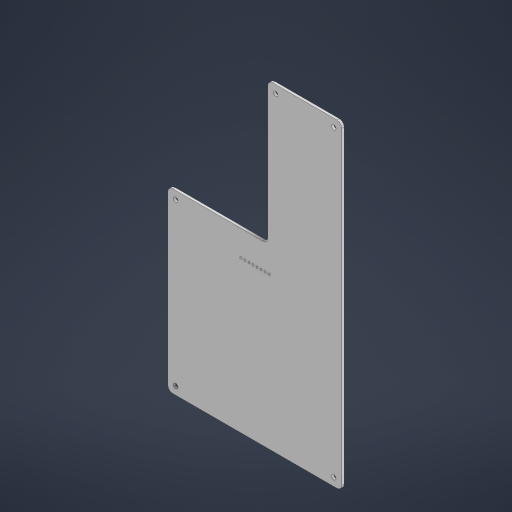
# Autodesk Inventor part: Motherboard
Saved by Autodesk Inventor 2023 (Build 270158000, 158)
## iProperties
Created: 2023-07-12
Part Number: Motherboard
Material: Типовые
Document SubType Name: Modeling
Designer: khrip
Density: 1 g/cm^3
Appearance: По умолчанию
Author: khrip
Autodesk Inventor part; units mm, degrees
ref_plane "YZ Plane" through (0, 0, 0) normal (1, 0, 0) x (0, 1, 0)
ref_plane "XZ Plane" through (0, 0, 0) normal (0, 1, 0) x (-1, 0, 0)
ref_plane "XY Plane" through (0, 0, 0) normal (0, 0, 1) x (1, 0, 0)
ref_plane "РабПлоскость1" through (0, 0, 0) normal (0, 0, 1) x (1, 0, 0)
ref_plane "РабПлоскость2" through (0, 0, 0) normal (0, 0, 1) x (1, 0, 0)
sketch "Эскиз2" plane through (0, 0, 0) normal (0, 0, 1) x (1, 0, 0)
  line L0 (164.5082, 55.3787) -> (164.5082, 22.6213)
  line L1 (152.0082, 55.3787) -> (164.5082, 55.3787)
  spline S0 degree 4 poles (142.0082, 66.7804) (141.9936, 65.5806) (142.2897, 63.8407) (143.0904, 61.8123) (144.7867, 59.6039) (146.7684, 57.7973) (148.9036, 56.5519) (150.6395, 55.9298) (152.0082, 55.3787) knots 0 0 0 0 0 0.305903 0.428365 0.551581 0.676311 1 1 1 1 1
  line L2 (142.0082, 89.6988) -> (142.0082, 66.7804)
  spline S1 degree 4 poles (142.0976, 90.5077) (142.1863, 90.3272) (142.1406, 90.1079) (142.065, 89.9075) (142.0082, 89.6988) knots 0 0 0 0 0 1 1 1 1 1
  ellipse E0 centre (144.0082, 89.6716) end of major axis (144.0082, 92.5) minor radius 2 (144.0082, 92.5) -> (142.0976, 90.5077) ccw
  line L3 (144.0082, 92.5) -> (149.4338, 92.5)
  line L4 (149.4338, 92.5) -> (149.4338, 92.525)
  line L5 (149.4338, 92.525) -> (142.946, 92.525)
  ellipse E1 centre (142.946, 98.525) end of major axis (136.7344, 98.525) minor radius 6 (136.7344, 98.525) -> (142.946, 92.525) ccw
  line L6 (136.7344, 98.525) -> (136.7344, 100.025)
  ellipse E2 centre (142.946, 100.025) end of major axis (136.7344, 100.025) minor radius 6 (142.946, 106.025) -> (136.7344, 100.025) ccw
  line L7 (142.946, 106.025) -> (149.4338, 106.025)
  line L8 (149.4338, 106.025) -> (149.4338, 106.05)
  line L9 (149.4338, 106.05) -> (144.0082, 106.05)
  ellipse E3 centre (144.0082, 108.8784) end of major axis (144.0082, 106.05) minor radius 2 (142.0976, 108.0423) -> (144.0082, 106.05) ccw
  spline S2 degree 4 poles (142.0082, 108.8512) (142.0222, 108.6489) (142.0418, 108.4466) (142.067, 108.2444) (142.0976, 108.0423) knots 0 0 0 0 0 1 1 1 1 1
  line L10 (142.0082, 108.8512) -> (142.0082, 139)
  arc A0 (142.0082, 139) -> (137.0082, 144) centre (137.0082, 139) ccw
  line L11 (137.0082, 144) -> (27.0082, 144)
  arc A1 (27.0082, 144) -> (22.0082, 139) centre (27.0082, 139) ccw
  line L12 (22.0082, 139) -> (22.0082, 108.8512)
  spline S3 degree 4 poles (21.9188, 108.0423) (21.9596, 108.2417) (21.9876, 108.4433) (22.0035, 108.6467) (22.0082, 108.8512) knots 0 0 0 0 0 1 1 1 1 1
  ellipse E4 centre (20.0082, 108.8784) end of major axis (20.0082, 106.05) minor radius 2 (20.0082, 106.05) -> (21.9188, 108.0423) ccw
  line L13 (14.5826, 106.05) -> (20.0082, 106.05)
  line L14 (14.5826, 106.025) -> (14.5826, 106.05)
  line L15 (21.0704, 106.025) -> (14.5826, 106.025)
  ellipse E5 centre (21.0704, 100.025) end of major axis (27.282, 100.025) minor radius 6 (27.282, 100.025) -> (21.0704, 106.025) ccw
  ellipse E6 centre (21.0704, 98.525) end of major axis (27.282, 98.525) minor radius 6 (21.0704, 92.525) -> (27.282, 98.525) ccw
  line L16 (14.5826, 92.525) -> (21.0704, 92.525)
  line L17 (14.5826, 92.5) -> (14.5826, 92.525)
  line L18 (20.0082, 92.5) -> (14.5826, 92.5)
  ellipse E7 centre (20.0082, 89.6716) end of major axis (20.0082, 92.5) minor radius 2 (21.9188, 90.5077) -> (20.0082, 92.5) ccw
  spline S4 degree 4 poles (22.0082, 89.6988) (22.0001, 89.9001) (21.9823, 90.1037) (21.9553, 90.3071) (21.9188, 90.5077) knots 0 0 0 0 0 1 1 1 1 1
  line L19 (22.0082, 89.6988) -> (22.0082, 66.7804)
  spline S5 degree 4 poles (12.0082, 55.3787) (13.3543, 55.9133) (15.0972, 56.5843) (17.1914, 57.7632) (19.2093, 59.6353) (20.8508, 61.7502) (21.742, 63.9004) (21.9889, 65.5297) (22.0082, 66.7804) knots 0 0 0 0 0 0.323057 0.447569 0.570948 0.693515 1 1 1 1 1
  line L20 (-0.4918, 55.3787) -> (12.0082, 55.3787)
  line L21 (-0.4918, 22.6213) -> (-0.4918, 55.3787)
  line L22 (12.0082, 22.6213) -> (-0.4918, 22.6213)
  spline S6 degree 4 poles (22.0082, 11.2196) (21.9907, 12.4712) (21.7455, 14.1022) (20.8556, 16.2534) (19.2129, 18.3699) (17.1941, 20.2411) (15.0987, 21.4185) (13.3552, 22.0877) (12.0082, 22.6213) knots 0 0 0 0 0 0.306528 0.4291 0.552475 0.676977 1 1 1 1 1
  line L23 (22.0082, -11.6988) -> (22.0082, 11.2196)
  spline S7 degree 4 poles (22.2969, -12.5077) (22.2375, -12.3039) (22.1691, -12.101) (22.0924, -11.8993) (22.0082, -11.6988) knots 0 0 0 0 0 1 1 1 1 1
  ellipse E8 centre (20.3863, -11.6716) end of major axis (20.3863, -14.5) minor radius 2 (20.3863, -14.5) -> (22.2969, -12.5077) ccw
  line L24 (20.3863, -14.5) -> (14.9607, -14.5)
  line L25 (14.9607, -14.5) -> (14.9607, -14.525)
  line L26 (14.9607, -14.525) -> (21.4484, -14.525)
  ellipse E9 centre (21.4484, -20.525) end of major axis (27.6601, -20.525) minor radius 6 (27.6601, -20.525) -> (21.4484, -14.525) ccw
  line L27 (27.6601, -20.525) -> (27.6601, -22.025)
  ellipse E10 centre (21.4484, -22.025) end of major axis (27.6601, -22.025) minor radius 6 (21.4484, -28.025) -> (27.6601, -22.025) ccw
  line L28 (21.4484, -28.025) -> (14.9607, -28.025)
  line L29 (14.9607, -28.025) -> (14.9607, -28.05)
  line L30 (14.9607, -28.05) -> (20.3863, -28.05)
  ellipse E11 centre (20.3863, -30.8784) end of major axis (20.3863, -28.05) minor radius 2 (22.2969, -30.0423) -> (20.3863, -28.05) ccw
  spline S8 degree 4 poles (22.0082, -30.8512) (22.0994, -30.6437) (22.1874, -30.4372) (22.2667, -30.2332) (22.2969, -30.0423) knots 0 0 0 0 0 1 1 1 1 1
  line L31 (22.0082, -30.8512) -> (22.0082, -61)
  arc A2 (22.0082, -61) -> (27.0082, -66) centre (27.0082, -61) ccw
  line L32 (27.0082, -66) -> (137.0082, -66)
  arc A3 (137.0082, -66) -> (142.0082, -61) centre (137.0082, -61) ccw
  line L33 (142.0082, -61) -> (142.0082, -30.8512)
  spline S9 degree 4 poles (142.0976, -30.0423) (142.0618, -30.2424) (142.0345, -30.444) (142.0164, -30.6471) (142.0082, -30.8512) knots 0 0 0 0 0 1 1 1 1 1
  ellipse E12 centre (144.0082, -30.8784) end of major axis (144.0082, -28.05) minor radius 2 (144.0082, -28.05) -> (142.0976, -30.0423) ccw
  line L34 (149.4338, -28.05) -> (144.0082, -28.05)
  line L35 (149.4338, -28.025) -> (149.4338, -28.05)
  line L36 (142.946, -28.025) -> (149.4338, -28.025)
  ellipse E13 centre (142.946, -22.025) end of major axis (136.7344, -22.025) minor radius 6 (136.7344, -22.025) -> (142.946, -28.025) ccw
  line L37 (136.7344, -20.525) -> (136.7344, -22.025)
  ellipse E14 centre (142.946, -20.525) end of major axis (136.7344, -20.525) minor radius 6 (142.0082, -14.5938) -> (136.7344, -20.525) ccw
  spline S10 degree 4 poles (143.3575, -14.5382) (143.017, -14.5392) (142.6788, -14.5494) (142.3414, -14.5663) (142.0082, -14.5938) knots 0 0 0 0 0 1 1 1 1 1
  spline S11 degree 4 poles (143.3575, -14.5382) (143.1143, -14.3292) (142.8382, -14.0321) (142.6629, -13.7922) (142.4735, -13.4852) knots 0 0 0 0 0 1 1 1 1 1
  ellipse E15 centre (144.0082, -11.6716) end of major axis (144.0082, -8.8431) minor radius 2 (142.0976, -12.5077) -> (142.4735, -13.4852) ccw
  spline S12 degree 4 poles (142.0976, -12.5077) (142.0566, -12.3073) (142.0277, -12.1043) (142.0113, -11.9008) (142.0082, -11.6988) knots 0 0 0 0 0 1 1 1 1 1
  line L38 (142.0082, 11.2196) -> (142.0082, -11.6988)
  spline S13 degree 4 poles (152.0082, 22.6213) (150.6678, 22.0949) (148.9359, 21.4381) (146.8415, 20.2599) (144.8098, 18.3825) (143.1469, 16.2574) (142.2323, 14.098) (142.0013, 12.4654) (142.0082, 11.2196) knots 0 0 0 0 0 0.322163 0.446837 0.570623 0.693583 1 1 1 1 1
  line L39 (164.5082, 22.6213) -> (152.0082, 22.6213)
  line L40 (27.282, 98.525) -> (27.282, 100.025)
  line L41 (27.6601, -66) -> (136.7344, -66)
  line L42 (136.7344, -66) -> (136.7344, 55.12)
  line L43 (85.3082, 55.12) -> (27.6601, 55.12)
  line L44 (27.6601, 55.12) -> (27.6601, -66)
  line L45 (49.6082, 55.12) -> (60.6082, 55.12) projected
  line L46 (85.3082, 55.12) -> (85.3082, 144)
  line L47 (85.3082, 144) -> (136.7344, 144)
  line L48 (136.7344, 144) -> (136.7344, 55.12)
  line L49 (85.3082, 113.52) -> (85.3082, 107.52) projected
  line L50 (84.3244, 70.87) -> (84.3244, 64.87) projected
  line L51 (27.6601, 50.12) -> (90.3082, 50.12)
  line L52 (136.7344, 57.0858) -> (136.7344, -61)
  line L53 (136.7344, -61) -> (27.6601, -61)
  line L54 (27.6601, -61) -> (27.6601, 50.12)
  line L55 (90.3082, 50.12) -> (90.3082, 139)
  line L56 (90.3082, 139) -> (136.7344, 139)
  line L57 (136.7344, 139) -> (136.7344, 57.0858)
  point P0 (0, 0)
  point P1 (142.0243, 108.6495)
  point P2 (142.0445, 108.4475)
  point P3 (142.069, 108.2451)
  point P4 (21.9548, 108.2422)
  point P5 (21.9815, 108.4436)
  point P6 (21.9992, 108.6466)
  point P7 (21.9966, 89.8995)
  point P8 (21.9778, 90.1023)
  point P9 (21.9518, 90.3056)
  point P10 (14.1516, 56.2573)
  point P11 (16.0588, 57.2184)
  point P12 (17.7454, 58.3637)
  point P13 (19.1678, 59.6884)
  point P14 (20.3459, 61.2222)
  point P15 (21.2579, 62.9881)
  point P16 (21.8122, 64.8416)
  point P17 (21.8145, 13.1602)
  point P18 (21.2616, 15.0151)
  point P19 (20.35, 16.7819)
  point P20 (19.1713, 18.3166)
  point P21 (17.7482, 19.6409)
  point P22 (16.0609, 20.785)
  point P23 (14.1529, 21.7445)
  point P24 (22.2348, -12.3061)
  point P25 (22.1658, -12.104)
  point P26 (22.0903, -11.9016)
  point P27 (22.102, -30.634)
  point P28 (22.1869, -30.423)
  point P29 (22.2547, -30.224)
  point P30 (142.0651, -30.2427)
  point P31 (142.0392, -30.4442)
  point P32 (142.0201, -30.6471)
  point P33 (143.0157, -14.5425)
  point P34 (142.6767, -14.5533)
  point P35 (142.3406, -14.5702)
  point P36 (143.1122, -14.3072)
  point P37 (142.8714, -14.0419)
  point P38 (142.6642, -13.7743)
  point P39 (142.061, -12.3056)
  point P40 (142.0338, -12.1027)
  point P41 (142.0162, -11.9001)
  point P42 (149.8807, 21.759)
  point P43 (147.9821, 20.8085)
  point P44 (146.2898, 19.6634)
  point P45 (144.8524, 18.3311)
  point P46 (143.6547, 16.7844)
  point P47 (142.7262, 15.0053)
  point P48 (142.1752, 13.1484)
  point P49 (142.1418, 90.326)
  point P50 (142.1248, 90.1256)
  point P51 (142.0712, 89.914)
  point P52 (142.1871, 64.8545)
  point P53 (142.7332, 62.9853)
  point P54 (143.6182, 61.2481)
  point P55 (144.8211, 59.6733)
  point P56 (146.2281, 58.3691)
  point P57 (147.919, 57.2204)
  point P58 (149.8389, 56.2585)
  point P59 (82.0082, 39)
  point P60 (136.7344, -21.275)
  point P61 (27.6601, -21.275)
  dimension "d5" = 0
  dimension "d6" = 0
  dimension "d7" = 0
  dimension "d8" = 0
  dimension "d9" = 0
  dimension "d10" = 5
  dimension "d11" = 5
  dimension "d12" = 0
  dimension "d13" = 5
  dimension "d14" = 0
  dimension "d15" = 5
  constraints: 110 end point, 9 horizontal, 8 point on circle, 7 vertical, 6 parallel, 4 centre point, 2 midpoint, 2 perpendicular, 1 point on line, 192 other
  measures "d5" distance from line of point (136.734, -21.275) L42
  measures "d6" distance from line of L44 point (27.66, -21.275)
  measures "d7" distance between parallel lines of L32 L41
  measures "d8" distance between parallel lines of L45 L43
  measures "d9" distance between parallel lines of L49 L46
  measures "d10" distance between parallel lines of L47 L56
  measures "d11" distance between parallel lines of L46 L55
  measures "d12" distance between parallel lines of L48 L57
  measures "d13" distance between parallel lines of L43 L51
  measures "d14" distance between parallel lines of L54 L44
  measures "d15" distance between parallel lines of L32 L53
extrude "Выдавливание1" add sketch "Эскиз2" along normal blind 1.5 contours L37 L42 L53 L44 L27 L51 L55 L56 L48 L6
fillet "Сопряжение1" radius 3 6 edges at (27.6601, 50.12, 0.75) (90.3082, 50.12, 0.75) (90.3082, 139, 0.75) (136.7344, 139, 0.75) (136.7344, -61, 0.75) (27.6601, -61, 0.75)
sketch "Эскиз3" plane through (0, 0, 1.5) normal (0, 0, 1) x (1, 0, 0)
  arc A0 (27.6601, -58) -> (30.6601, -61) centre (30.6601, -58) ccw projected
  line L0 (30.6601, -61) -> (133.7344, -61) projected
  arc A1 (133.7344, -61) -> (136.7344, -58) centre (133.7344, -58) ccw projected
  line L1 (136.7344, -58) -> (136.7344, 136) projected
  arc A2 (136.7344, 136) -> (133.7344, 139) centre (133.7344, 136) ccw projected
  line L2 (133.7344, 139) -> (93.3082, 139) projected
  arc A3 (93.3082, 139) -> (90.3082, 136) centre (93.3082, 136) ccw projected
  line L3 (90.3082, 136) -> (90.3082, 53.12) projected
  arc A4 (87.3082, 50.12) -> (90.3082, 53.12) centre (87.3082, 53.12) ccw projected
  line L4 (87.3082, 50.12) -> (30.6601, 50.12) projected
  arc A5 (30.6601, 50.12) -> (27.6601, 47.12) centre (30.6601, 47.12) ccw projected
  line L5 (27.6601, 47.12) -> (27.6601, -58) projected
  circle A6 centre (32.6601, -56) radius 1.5
  circle A7 centre (32.6601, 45.12) radius 1.5
  circle A8 centre (131.7344, -56) radius 1.5
  circle A9 centre (131.7344, 134) radius 1.5
  circle A10 centre (95.3082, 134) radius 1.5
  point P0 (0, 0)
  dimension "d19" = 5
  dimension "d20" = 3
  dimension "d21" = 5
  dimension "d22" = 3
  dimension "d23" = 3
  dimension "d24" = 3
  dimension "d25" = 3
  dimension "d26" = 5
  dimension "d27" = 5
  dimension "d28" = 5
  dimension "d29" = 5
  dimension "d30" = 5
  dimension "d31" = 5
  dimension "d32" = 5
  dimension "d33" = 5
  constraints: 5 centre point
  measures "d19" distance from line of L0 A6.centre
  measures "d20" diameter of A6
  measures "d21" distance from line of L5 A6.centre
  measures "d22" diameter of A7
  measures "d23" diameter of A8
  measures "d24" diameter of A9
  measures "d25" diameter of A10
  measures "d26" distance from line of L2 A10.centre
  measures "d27" distance from line of L3 A10.centre
  measures "d28" distance from line of L1 A9.centre
  measures "d29" distance from line of L2 A9.centre
  measures "d30" distance from line of L0 A8.centre
  measures "d31" distance from line of L1 A8.centre
  measures "d32" distance from line of L5 A7.centre
  measures "d33" distance from line of L4 A7.centre
hole "Отверстие1" at (32.6601, 45.12, 1.5) at (32.6601, -56, 1.5) at (131.7344, -56, 1.5) at (131.7344, 134, 1.5) at (95.3082, 134, 1.5) direction (0, 0, -1) diameter 2.9 end through all clearance for "Винт с потайной головкой ISO 2009/7046" size "M2.5" standard "ISO"
sketch "Эскиз4" plane through (0, 0, 1.5) normal (0, 0, 1) x (1, 0, 0)
  circle A0 centre (73.4444, 34) radius 0.6 projected
  circle A1 centre (75.9844, 34) radius 0.6 projected
  circle A2 centre (78.5244, 34) radius 0.6 projected
  circle A3 centre (81.0644, 34) radius 0.6 projected
  circle A4 centre (83.6044, 34) radius 0.6 projected
  circle A5 centre (86.1444, 34) radius 0.6 projected
  circle A6 centre (88.6844, 34) radius 0.6 projected
  circle A7 centre (91.2244, 34) radius 0.6 projected
  point P0 (0, 0)
extrude "Выдавливание2" cut sketch "Эскиз4" against normal blind 10
